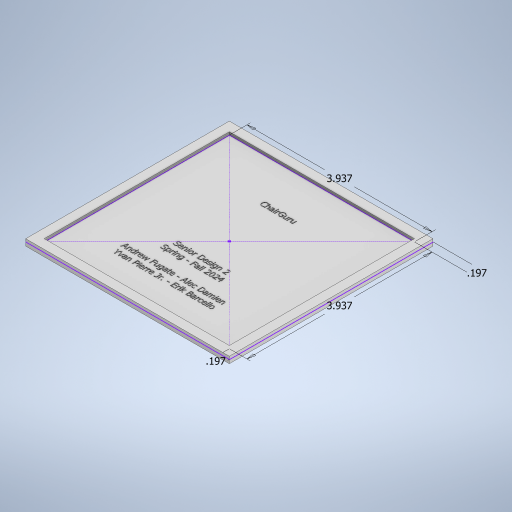
# Autodesk Inventor part: BumperCustomPCB
Saved by Autodesk Inventor 2023 (Build 270158000, 158)
## iProperties
Created: 2024-11-15
Part Number: BumperCustomPCB
Material: Generic
Document SubType Name: Modeling
Designer: andre
Density: 1 g/cm^3
Appearance: Default
Author: andre
Autodesk Inventor part; units mm, degrees
(part 1 of 3)
ref_plane "YZ Plane" through (0, 0, 0) normal (1, 0, 0) x (0, 1, 0)
ref_plane "XZ Plane" through (0, 0, 0) normal (0, 1, 0) x (-1, 0, 0)
ref_plane "XY Plane" through (0, 0, 0) normal (0, 0, 1) x (1, 0, 0)
sketch "Sketch1" plane through (0, 0, 0) normal (0, 1, 0) x (-1, 0, 0)
  line L0 (50, 50) -> (-50, 50)
  line L1 (-50, 50) -> (-50, -50)
  line L2 (-50, -50) -> (50, -50)
  line L3 (50, -50) -> (50, 50)
  line L4 (50, 50) -> (-50, -50) construction
  line L5 (-50, 50) -> (50, -50) construction
  line L6 (55, 55) -> (-55, 55)
  line L7 (-55, 55) -> (-55, -55)
  line L8 (-55, -55) -> (55, -55)
  line L9 (55, -55) -> (55, 55)
  line L10 (55, 55) -> (-55, -55) construction
  line L11 (-55, 55) -> (55, -55) construction
  point P0 (0, 0)
  dimension "d1" = 100
  dimension "d2" = 100
  dimension "d3" = 5
  dimension "d4" = 5
  constraints: 24 end point, 4 midpoint, 4 parallel, 2 horizontal, 2 perpendicular
  measures "d1" distance of L2.end L1.end
  measures "d2" distance of L1.end L0.end
  measures "d3" distance between parallel lines of L2 L8
  measures "d4" distance between parallel lines of L7 L1
extrude "Extrusion1" add sketch "Sketch1" against normal blind 2 contours L3 L2 L1 L0
extrude "Extrusion4" add sketch "Sketch1" along normal blind 1.5
extrude "Extrusion5" add sketch "Sketch1" against normal blind 2 contours L3 L2 L1 L0 | L9 L8 L7 L6
sketch "Sketch2" plane through (0, 0, 0) normal (0, 1, 0) x (1, 0, 0)
  line L0 (-9.5845, 43.6431) -> (8.9233, 43.6431) construction
  line L1 (8.9233, 43.6431) -> (8.9233, 10.4968) construction
  line L2 (8.9233, 10.4968) -> (-9.5845, 10.4968) construction
  line L3 (-9.5845, 10.4968) -> (-9.5845, 43.6431) construction
  line L4 (-49.3127, 0.1016) -> (49.3774, 0.1016) construction
  line L5 (49.3774, 0.1016) -> (49.3774, -49.8419) construction
  line L6 (49.3774, -49.8419) -> (-49.3127, -49.8419) construction
  line L7 (-49.3127, -49.8419) -> (-49.3127, 0.1016) construction
  spline S0 degree 2 poles (-8.0852, 25.4558) (-8.3816, 25.4558) (-8.883, 25.6559) (-9.0658, 25.856) knots 0 0 0 1 2 2 2
  spline S1 degree 2 poles (-9.0658, 25.856) (-9.2486, 26.0536) (-9.4486, 26.6464) (-9.4486, 27.0317) knots 0 0 0 1 2 2 2
  spline S2 degree 2 poles (-9.4486, 27.0317) (-9.4486, 27.4145) (-9.2535, 27.9826) (-9.0683, 28.1926) knots 0 0 0 1 2 2 2
  spline S3 degree 2 poles (-9.0683, 28.1926) (-8.8855, 28.3976) (-8.3865, 28.6125) (-8.0778, 28.6125) knots 0 0 0 1 2 2 2
  spline S4 degree 2 poles (-8.0778, 28.6125) (-7.9246, 28.6125) (-7.6554, 28.568) (-7.5418, 28.5335) knots 0 0 0 1 2 2 2
  spline S5 degree 2 poles (-7.5418, 28.5335) (-7.443, 28.5013) (-7.238, 28.41) (-7.1367, 28.3556) knots 0 0 0 1 2 2 2
  line L8 (-7.1367, 28.3556) -> (-7.1367, 27.8666)
  line L9 (-7.1367, 27.8666) -> (-7.1688, 27.8666)
  spline S6 degree 2 poles (-7.1688, 27.8666) (-7.2231, 27.916) (-7.3911, 28.0543) (-7.5121, 28.121) knots 0 0 0 1 2 2 2
  spline S7 degree 2 poles (-7.5121, 28.121) (-7.6282, 28.1852) (-7.9024, 28.2667) (-8.0802, 28.2667) knots 0 0 0 1 2 2 2
  spline S8 degree 2 poles (-8.0802, 28.2667) (-8.2754, 28.2667) (-8.6236, 28.1061) (-8.7546, 27.953) knots 0 0 0 1 2 2 2
  spline S9 degree 2 poles (-8.7546, 27.953) (-8.883, 27.7974) (-9.0263, 27.3256) (-9.0263, 27.0317) knots 0 0 0 1 2 2 2
  spline S10 degree 2 poles (-9.0263, 27.0317) (-9.0263, 26.718) (-8.8756, 26.266) (-8.7447, 26.1104) knots 0 0 0 1 2 2 2
  spline S11 degree 2 poles (-8.7447, 26.1104) (-8.6162, 25.9597) (-8.2729, 25.8066) (-8.0802, 25.8066) knots 0 0 0 1 2 2 2
  spline S12 degree 2 poles (-8.0802, 25.8066) (-7.9049, 25.8066) (-7.606, 25.893) (-7.4899, 25.9572) knots 0 0 0 1 2 2 2
  spline S13 degree 2 poles (-7.4899, 25.9572) (-7.3788, 26.0215) (-7.2133, 26.1548) (-7.1663, 26.2018) knots 0 0 0 1 2 2 2
  line L10 (-7.1663, 26.2018) -> (-7.1367, 26.2018)
  line L11 (-7.1367, 26.2018) -> (-7.1367, 25.7176)
  spline S14 degree 2 poles (-7.1367, 25.7176) (-7.238, 25.6707) (-7.4158, 25.5843) (-7.5418, 25.5447) knots 0 0 0 1 2 2 2
  spline S15 degree 2 poles (-7.5418, 25.5447) (-7.6752, 25.5003) (-7.9024, 25.4558) (-8.0852, 25.4558) knots 0 0 0 1 2 2 2
  line L12 (-4.9927, 25.5102) -> (-5.378, 25.5102)
  line L13 (-5.378, 25.5102) -> (-5.378, 26.8143)
  spline S16 degree 2 poles (-5.378, 26.8143) (-5.378, 26.9724) (-5.4077, 27.2441) (-5.4521, 27.3256) knots 0 0 0 1 2 2 2
  spline S17 degree 2 poles (-5.4521, 27.3256) (-5.4991, 27.4121) (-5.667, 27.4961) (-5.8103, 27.4961) knots 0 0 0 1 2 2 2
  spline S18 degree 2 poles (-5.8103, 27.4961) (-5.9536, 27.4961) (-6.2574, 27.3429) (-6.4031, 27.2194) knots 0 0 0 1 2 2 2
  line L14 (-6.4031, 27.2194) -> (-6.4031, 25.5102)
  line L15 (-6.4031, 25.5102) -> (-6.7884, 25.5102)
  line L16 (-6.7884, 25.5102) -> (-6.7884, 28.694)
  line L17 (-6.7884, 28.694) -> (-6.4031, 28.694)
  line L18 (-6.4031, 28.694) -> (-6.4031, 27.543)
  spline S19 degree 2 poles (-6.4031, 27.543) (-6.2302, 27.6986) (-5.8968, 27.8616) (-5.709, 27.8616) knots 0 0 0 1 2 2 2
  spline S20 degree 2 poles (-5.709, 27.8616) (-5.3731, 27.8616) (-4.9927, 27.417) (-4.9927, 26.9946) knots 0 0 0 1 2 2 2
  line L19 (-4.9927, 26.9946) -> (-4.9927, 25.5102)
  spline S21 degree 2 poles (-3.1773, 25.7522) (-3.2242, 25.7176) (-3.3823, 25.5941) (-3.4564, 25.5571) knots 0 0 0 1 2 2 2
  spline S22 degree 2 poles (-3.4564, 25.5571) (-3.5576, 25.5027) (-3.7478, 25.4459) (-3.9207, 25.4459) knots 0 0 0 1 2 2 2
  spline S23 degree 2 poles (-3.9207, 25.4459) (-4.0615, 25.4459) (-4.3159, 25.5521) (-4.4123, 25.6485) knots 0 0 0 1 2 2 2
  spline S24 degree 2 poles (-4.4123, 25.6485) (-4.5037, 25.7423) (-4.6148, 26.019) (-4.6148, 26.1721) knots 0 0 0 1 2 2 2
  spline S25 degree 2 poles (-4.6148, 26.1721) (-4.6148, 26.4092) (-4.4147, 26.7452) (-4.1974, 26.8415) knots 0 0 0 1 2 2 2
  spline S26 degree 2 poles (-4.1974, 26.8415) (-4.0047, 26.9304) (-3.4811, 26.9971) (-3.1773, 27.0144) knots 0 0 0 1 2 2 2
  line L20 (-3.1773, 27.0144) -> (-3.1773, 27.0885)
  spline S27 degree 2 poles (-3.1773, 27.0885) (-3.1773, 27.2219) (-3.2588, 27.3874) (-3.3329, 27.4343) knots 0 0 0 1 2 2 2
  spline S28 degree 2 poles (-3.3329, 27.4343) (-3.407, 27.4812) (-3.6194, 27.5109) (-3.733, 27.5109) knots 0 0 0 1 2 2 2
  spline S29 degree 2 poles (-3.733, 27.5109) (-3.8664, 27.5109) (-4.227, 27.4318) (-4.4073, 27.3553) knots 0 0 0 1 2 2 2
  line L21 (-4.4073, 27.3553) -> (-4.4296, 27.3553)
  line L22 (-4.4296, 27.3553) -> (-4.4296, 27.748)
  spline S30 degree 2 poles (-4.4296, 27.748) (-4.3234, 27.7776) (-3.9257, 27.8517) (-3.7305, 27.8517) knots 0 0 0 1 2 2 2
  spline S31 degree 2 poles (-3.7305, 27.8517) (-3.4934, 27.8517) (-3.1699, 27.7776) (-3.0414, 27.6813) knots 0 0 0 1 2 2 2
  spline S32 degree 2 poles (-3.0414, 27.6813) (-2.9154, 27.5874) (-2.7919, 27.2886) (-2.7919, 27.0737) knots 0 0 0 1 2 2 2
  line L23 (-2.7919, 27.0737) -> (-2.7919, 25.5102)
  line L24 (-2.7919, 25.5102) -> (-3.1773, 25.5102)
  line L25 (-3.1773, 25.5102) -> (-3.1773, 25.7522)
  line L26 (-3.1773, 26.0733) -> (-3.1773, 26.7081)
  spline S33 degree 2 poles (-3.1773, 26.7081) (-3.3156, 26.6958) (-3.733, 26.6538) (-3.8639, 26.6143) knots 0 0 0 1 2 2 2
  spline S34 degree 2 poles (-3.8639, 26.6143) (-4.0171, 26.5673) (-4.2171, 26.3722) (-4.2171, 26.1993) knots 0 0 0 1 2 2 2
  spline S35 degree 2 poles (-4.2171, 26.1993) (-4.2171, 26.0017) (-3.9948, 25.8016) (-3.7824, 25.8016) knots 0 0 0 1 2 2 2
  spline S36 degree 2 poles (-3.7824, 25.8016) (-3.6021, 25.8016) (-3.3057, 25.9572) (-3.1773, 26.0733) knots 0 0 0 1 2 2 2
  line L27 (-1.8583, 25.5102) -> (-2.2436, 25.5102)
  line L28 (-2.2436, 25.5102) -> (-2.2436, 27.7974)
  line L29 (-2.2436, 27.7974) -> (-1.8583, 27.7974)
  line L30 (-1.8583, 27.7974) -> (-1.8583, 25.5102)
  line L31 (-1.8311, 28.1778) -> (-2.2683, 28.1778)
  line L32 (-2.2683, 28.1778) -> (-2.2683, 28.5779)
  line L33 (-2.2683, 28.5779) -> (-1.8311, 28.5779)
  line L34 (-1.8311, 28.5779) -> (-1.8311, 28.1778)
  line L35 (-0.0799, 27.3849) -> (-0.0996, 27.3849)
  spline S37 degree 2 poles (-0.0996, 27.3849) (-0.1441, 27.3973) (-0.2404, 27.4022) (-0.3071, 27.4022) knots 0 0 0 1 2 2 2
  spline S38 degree 2 poles (-0.3071, 27.4022) (-0.4627, 27.4022) (-0.769, 27.2663) (-0.9073, 27.133) knots 0 0 0 1 2 2 2
  line L36 (-0.9073, 27.133) -> (-0.9073, 25.5102)
  line L37 (-0.9073, 25.5102) -> (-1.2926, 25.5102)
  line L38 (-1.2926, 25.5102) -> (-1.2926, 27.7974)
  line L39 (-1.2926, 27.7974) -> (-0.9073, 27.7974)
  line L40 (-0.9073, 27.7974) -> (-0.9073, 27.4565)
  spline S39 degree 2 poles (-0.9073, 27.4565) (-0.6974, 27.6443) (-0.3837, 27.7974) (-0.2355, 27.7974) knots 0 0 0 1 2 2 2
  spline S40 degree 2 poles (-0.2355, 27.7974) (-0.1762, 27.7974) (-0.1169, 27.7925) (-0.0799, 27.785) knots 0 0 0 1 2 2 2
  line L41 (-0.0799, 27.785) -> (-0.0799, 27.3849)
  spline S41 degree 2 poles (1.5256, 25.4509) (1.2021, 25.4509) (0.6661, 25.6485) (0.4734, 25.8486) knots 0 0 0 1 2 2 2
  spline S42 degree 2 poles (0.4734, 25.8486) (0.2808, 26.0511) (0.0757, 26.6488) (0.0757, 27.0366) knots 0 0 0 1 2 2 2
  spline S43 degree 2 poles (0.0757, 27.0366) (0.0757, 27.4047) (0.2832, 27.9876) (0.4759, 28.1951) knots 0 0 0 1 2 2 2
  spline S44 degree 2 poles (0.4759, 28.1951) (0.6611, 28.3951) (1.2045, 28.6125) (1.5281, 28.6125) knots 0 0 0 1 2 2 2
  spline S45 degree 2 poles (1.5281, 28.6125) (1.6837, 28.6125) (1.9653, 28.568) (2.0938, 28.5285) knots 0 0 0 1 2 2 2
  spline S46 degree 2 poles (2.0938, 28.5285) (2.1975, 28.4989) (2.4494, 28.3902) (2.526, 28.3507) knots 0 0 0 1 2 2 2
  line L42 (2.526, 28.3507) -> (2.526, 27.8616)
  line L43 (2.526, 27.8616) -> (2.4914, 27.8616)
  spline S47 degree 2 poles (2.4914, 27.8616) (2.4149, 27.9283) (2.2543, 28.0493) (2.1061, 28.1185) knots 0 0 0 1 2 2 2
  spline S48 degree 2 poles (2.1061, 28.1185) (1.9826, 28.1802) (1.664, 28.2618) (1.4812, 28.2618) knots 0 0 0 1 2 2 2
  spline S49 degree 2 poles (1.4812, 28.2618) (1.0415, 28.2618) (0.4981, 27.5998) (0.4981, 27.049) knots 0 0 0 1 2 2 2
  spline S50 degree 2 poles (0.4981, 27.049) (0.4981, 26.7427) (0.6414, 26.2833) (0.7772, 26.1252) knots 0 0 0 1 2 2 2
  spline S51 degree 2 poles (0.7772, 26.1252) (0.9081, 25.9671) (1.2786, 25.8016) (1.5108, 25.8016) knots 0 0 0 1 2 2 2
  spline S52 degree 2 poles (1.5108, 25.8016) (1.6813, 25.8016) (2.0221, 25.851) (2.1382, 25.9004) knots 0 0 0 1 2 2 2
  line L44 (2.1382, 25.9004) -> (2.1382, 26.6884)
  line L45 (2.1382, 26.6884) -> (1.4318, 26.6884)
  line L46 (1.4318, 26.6884) -> (1.4318, 27.044)
  line L47 (1.4318, 27.044) -> (2.5384, 27.044)
  line L48 (2.5384, 27.044) -> (2.5384, 25.7127)
  spline S53 degree 2 poles (2.5384, 25.7127) (2.4618, 25.6781) (2.2, 25.5719) (2.0888, 25.5398) knots 0 0 0 1 2 2 2
  spline S54 degree 2 poles (2.0888, 25.5398) (1.9381, 25.4953) (1.6961, 25.4509) (1.5256, 25.4509) knots 0 0 0 1 2 2 2
  line L49 (4.7959, 25.5102) -> (4.4106, 25.5102)
  line L50 (4.4106, 25.5102) -> (4.4106, 25.7621)
  spline S55 degree 2 poles (4.4106, 25.7621) (4.2328, 25.6065) (3.9142, 25.4459) (3.7166, 25.4459) knots 0 0 0 1 2 2 2
  spline S56 degree 2 poles (3.7166, 25.4459) (3.5684, 25.4459) (3.3041, 25.5447) (3.2077, 25.6509) knots 0 0 0 1 2 2 2
  spline S57 degree 2 poles (3.2077, 25.6509) (3.1089, 25.7572) (3.0002, 26.0807) (3.0002, 26.3129) knots 0 0 0 1 2 2 2
  line L51 (3.0002, 26.3129) -> (3.0002, 27.7974)
  line L52 (3.0002, 27.7974) -> (3.3856, 27.7974)
  line L53 (3.3856, 27.7974) -> (3.3856, 26.4932)
  spline S58 degree 2 poles (3.3856, 26.4932) (3.3856, 26.3104) (3.4127, 26.0709) (3.4597, 25.9819) knots 0 0 0 1 2 2 2
  spline S59 degree 2 poles (3.4597, 25.9819) (3.5066, 25.893) (3.6672, 25.8115) (3.8178, 25.8115) knots 0 0 0 1 2 2 2
  spline S60 degree 2 poles (3.8178, 25.8115) (3.9586, 25.8115) (4.2772, 25.9721) (4.4106, 26.0881) knots 0 0 0 1 2 2 2
  line L54 (4.4106, 26.0881) -> (4.4106, 27.7974)
  line L55 (4.4106, 27.7974) -> (4.7959, 27.7974)
  line L56 (4.7959, 27.7974) -> (4.7959, 25.5102)
  line L57 (6.567, 27.3849) -> (6.5472, 27.3849)
  spline S61 degree 2 poles (6.5472, 27.3849) (6.5027, 27.3973) (6.4064, 27.4022) (6.3397, 27.4022) knots 0 0 0 1 2 2 2
  spline S62 degree 2 poles (6.3397, 27.4022) (6.1841, 27.4022) (5.8778, 27.2663) (5.7395, 27.133) knots 0 0 0 1 2 2 2
  line L58 (5.7395, 27.133) -> (5.7395, 25.5102)
  line L59 (5.7395, 25.5102) -> (5.3542, 25.5102)
  line L60 (5.3542, 25.5102) -> (5.3542, 27.7974)
  line L61 (5.3542, 27.7974) -> (5.7395, 27.7974)
  line L62 (5.7395, 27.7974) -> (5.7395, 27.4565)
  spline S63 degree 2 poles (5.7395, 27.4565) (5.9494, 27.6443) (6.2631, 27.7974) (6.4113, 27.7974) knots 0 0 0 1 2 2 2
  spline S64 degree 2 poles (6.4113, 27.7974) (6.4706, 27.7974) (6.5299, 27.7925) (6.567, 27.785) knots 0 0 0 1 2 2 2
  line L63 (6.567, 27.785) -> (6.567, 27.3849)
  line L64 (8.6442, 25.5102) -> (8.2589, 25.5102)
  line L65 (8.2589, 25.5102) -> (8.2589, 25.7621)
  spline S65 degree 2 poles (8.2589, 25.7621) (8.0811, 25.6065) (7.7624, 25.4459) (7.5648, 25.4459) knots 0 0 0 1 2 2 2
  spline S66 degree 2 poles (7.5648, 25.4459) (7.4166, 25.4459) (7.1523, 25.5447) (7.056, 25.6509) knots 0 0 0 1 2 2 2
  spline S67 degree 2 poles (7.056, 25.6509) (6.9572, 25.7572) (6.8485, 26.0807) (6.8485, 26.3129) knots 0 0 0 1 2 2 2
  line L66 (6.8485, 26.3129) -> (6.8485, 27.7974)
  line L67 (6.8485, 27.7974) -> (7.2339, 27.7974)
  line L68 (7.2339, 27.7974) -> (7.2339, 26.4932)
  spline S68 degree 2 poles (7.2339, 26.4932) (7.2339, 26.3104) (7.261, 26.0709) (7.308, 25.9819) knots 0 0 0 1 2 2 2
  spline S69 degree 2 poles (7.308, 25.9819) (7.3549, 25.893) (7.5154, 25.8115) (7.6661, 25.8115) knots 0 0 0 1 2 2 2
  spline S70 degree 2 poles (7.6661, 25.8115) (7.8069, 25.8115) (8.1255, 25.9721) (8.2589, 26.0881) knots 0 0 0 1 2 2 2
  line L69 (8.2589, 26.0881) -> (8.2589, 27.7974)
  line L70 (8.2589, 27.7974) -> (8.6442, 27.7974)
  line L71 (8.6442, 27.7974) -> (8.6442, 25.5102)
  spline S71 degree 2 poles (-13.3379, -16.4116) (-13.6688, -16.4116) (-14.1332, -16.2733) (-14.3382, -16.1745) knots 0 0 0 1 2 2 2
  line L72 (-14.3382, -16.1745) -> (-14.3382, -15.6657)
  line L73 (-14.3382, -15.6657) -> (-14.3086, -15.6657)
  spline S72 degree 2 poles (-14.3086, -15.6657) (-14.1085, -15.8534) (-13.6022, -16.0609) (-13.3675, -16.0609) knots 0 0 0 1 2 2 2
  spline S73 degree 2 poles (-13.3675, -16.0609) (-13.0316, -16.0609) (-12.6882, -15.7818) (-12.6882, -15.552) knots 0 0 0 1 2 2 2
  spline S74 degree 2 poles (-12.6882, -15.552) (-12.6882, -15.3693) (-12.8686, -15.142) (-13.0637, -15.0852) knots 0 0 0 1 2 2 2
  spline S75 degree 2 poles (-13.0637, -15.0852) (-13.2045, -15.0457) (-13.4391, -14.9914) (-13.6145, -14.9469) knots 0 0 0 1 2 2 2
  spline S76 degree 2 poles (-13.6145, -14.9469) (-13.7726, -14.9049) (-14.0221, -14.7789) (-14.1184, -14.6777) knots 0 0 0 1 2 2 2
  spline S77 degree 2 poles (-14.1184, -14.6777) (-14.2122, -14.5764) (-14.316, -14.3047) (-14.316, -14.1268) knots 0 0 0 1 2 2 2
  spline S78 degree 2 poles (-14.316, -14.1268) (-14.316, -13.7563) (-13.738, -13.2549) (-13.2909, -13.2549) knots 0 0 0 1 2 2 2
  spline S79 degree 2 poles (-13.2909, -13.2549) (-13.0341, -13.2549) (-12.5796, -13.3562) (-12.3844, -13.4525) knots 0 0 0 1 2 2 2
  line L74 (-12.3844, -13.4525) -> (-12.3844, -13.9367)
  line L75 (-12.3844, -13.9367) -> (-12.4141, -13.9367)
  spline S80 degree 2 poles (-12.4141, -13.9367) (-12.5598, -13.8033) (-13.0143, -13.6057) (-13.2638, -13.6057) knots 0 0 0 1 2 2 2
  spline S81 degree 2 poles (-13.2638, -13.6057) (-13.5453, -13.6057) (-13.8936, -13.87) (-13.8936, -14.0849) knots 0 0 0 1 2 2 2
  spline S82 degree 2 poles (-13.8936, -14.0849) (-13.8936, -14.2775) (-13.6886, -14.5072) (-13.4959, -14.5591) knots 0 0 0 1 2 2 2
  spline S83 degree 2 poles (-13.4959, -14.5591) (-13.3675, -14.5937) (-12.9945, -14.6826) (-12.871, -14.7197) knots 0 0 0 1 2 2 2
  spline S84 degree 2 poles (-12.871, -14.7197) (-12.5573, -14.816) (-12.2659, -15.2038) (-12.2659, -15.4878) knots 0 0 0 1 2 2 2
  spline S85 degree 2 poles (-12.2659, -15.4878) (-12.2659, -15.6681) (-12.4116, -16.0139) (-12.5425, -16.135) knots 0 0 0 1 2 2 2
  spline S86 degree 2 poles (-12.5425, -16.135) (-12.6882, -16.2684) (-13.0588, -16.4116) (-13.3379, -16.4116) knots 0 0 0 1 2 2 2
  spline S87 degree 2 poles (-10.8901, -16.4091) (-11.4384, -16.4091) (-12.0411, -15.7941) (-12.0411, -15.226) knots 0 0 0 1 2 2 2
  spline S88 degree 2 poles (-12.0411, -15.226) (-12.0411, -14.6678) (-11.4557, -14.0058) (-10.9839, -14.0058) knots 0 0 0 1 2 2 2
  spline S89 degree 2 poles (-10.9839, -14.0058) (-10.7715, -14.0058) (-10.443, -14.1293) (-10.322, -14.2602) knots 0 0 0 1 2 2 2
  spline S90 degree 2 poles (-10.322, -14.2602) (-10.1985, -14.3911) (-10.0676, -14.7691) (-10.0676, -15.0432) knots 0 0 0 1 2 2 2
  line L76 (-10.0676, -15.0432) -> (-10.0676, -15.2532)
  line L77 (-10.0676, -15.2532) -> (-11.6508, -15.2532)
  spline S91 degree 2 poles (-11.6508, -15.2532) (-11.6508, -15.6508) (-11.2507, -16.0732) (-10.895, -16.0732) knots 0 0 0 1 2 2 2
  spline S92 degree 2 poles (-10.895, -16.0732) (-10.769, -16.0732) (-10.5245, -16.0164) (-10.4257, -15.972) knots 0 0 0 1 2 2 2
  spline S93 degree 2 poles (-10.4257, -15.972) (-10.322, -15.9226) (-10.1787, -15.8361) (-10.1318, -15.7966) knots 0 0 0 1 2 2 2
  line L78 (-10.1318, -15.7966) -> (-10.1096, -15.7966)
  line L79 (-10.1096, -15.7966) -> (-10.1096, -16.2165)
  spline S94 degree 2 poles (-10.1096, -16.2165) (-10.1762, -16.2437) (-10.3788, -16.3227) (-10.4578, -16.3449) knots 0 0 0 1 2 2 2
  spline S95 degree 2 poles (-10.4578, -16.3449) (-10.569, -16.377) (-10.7518, -16.4091) (-10.8901, -16.4091) knots 0 0 0 1 2 2 2
  spline S96 degree 2 poles (-10.443, -14.9592) (-10.4479, -14.8036) (-10.5122, -14.5764) (-10.5739, -14.4998) knots 0 0 0 1 2 2 2
  spline S97 degree 2 poles (-10.5739, -14.4998) (-10.6406, -14.4134) (-10.8506, -14.322) (-11.0062, -14.322) knots 0 0 0 1 2 2 2
  spline S98 degree 2 poles (-11.0062, -14.322) (-11.1593, -14.322) (-11.3742, -14.4134) (-11.4631, -14.5023) knots 0 0 0 1 2 2 2
  spline S99 degree 2 poles (-11.4631, -14.5023) (-11.5496, -14.5937) (-11.6385, -14.8135) (-11.6508, -14.9592) knots 0 0 0 1 2 2 2
  line L80 (-11.6508, -14.9592) -> (-10.443, -14.9592)
  line L81 (-7.8816, -16.3573) -> (-8.2669, -16.3573)
  line L82 (-8.2669, -16.3573) -> (-8.2669, -15.0531)
  spline S100 degree 2 poles (-8.2669, -15.0531) (-8.2669, -14.895) (-8.2966, -14.6233) (-8.341, -14.5418) knots 0 0 0 1 2 2 2
  spline S101 degree 2 poles (-8.341, -14.5418) (-8.388, -14.4554) (-8.5559, -14.3714) (-8.6992, -14.3714) knots 0 0 0 1 2 2 2
  spline S102 degree 2 poles (-8.6992, -14.3714) (-8.8424, -14.3714) (-9.1462, -14.5245) (-9.292, -14.648) knots 0 0 0 1 2 2 2
  line L83 (-9.292, -14.648) -> (-9.292, -16.3573)
  line L84 (-9.292, -16.3573) -> (-9.6773, -16.3573)
  line L85 (-9.6773, -16.3573) -> (-9.6773, -14.07)
  line L86 (-9.6773, -14.07) -> (-9.292, -14.07)
  line L87 (-9.292, -14.07) -> (-9.292, -14.3244)
  spline S103 degree 2 poles (-9.292, -14.3244) (-9.1191, -14.1688) (-8.7856, -14.0058) (-8.5979, -14.0058) knots 0 0 0 1 2 2 2
  spline S104 degree 2 poles (-8.5979, -14.0058) (-8.262, -14.0058) (-7.8816, -14.4504) (-7.8816, -14.8728) knots 0 0 0 1 2 2 2
  line L88 (-7.8816, -14.8728) -> (-7.8816, -16.3573)
  line L89 (-6.9479, -16.3573) -> (-7.3333, -16.3573)
  line L90 (-7.3333, -16.3573) -> (-7.3333, -14.07)
  line L91 (-7.3333, -14.07) -> (-6.9479, -14.07)
  line L92 (-6.9479, -14.07) -> (-6.9479, -16.3573)
  line L93 (-6.9208, -13.6897) -> (-7.358, -13.6897)
  line L94 (-7.358, -13.6897) -> (-7.358, -13.2895)
  line L95 (-7.358, -13.2895) -> (-6.9208, -13.2895)
  line L96 (-6.9208, -13.2895) -> (-6.9208, -13.6897)
  spline S105 degree 2 poles (-4.5026, -15.2137) (-4.5026, -15.7916) (-5.0584, -16.4215) (-5.5227, -16.4215) knots 0 0 0 1 2 2 2
  spline S106 degree 2 poles (-5.5227, -16.4215) (-5.9994, -16.4215) (-6.5453, -15.7719) (-6.5453, -15.2137) knots 0 0 0 1 2 2 2
  spline S107 degree 2 poles (-6.5453, -15.2137) (-6.5453, -14.6406) (-5.9822, -14.0058) (-5.5227, -14.0058) knots 0 0 0 1 2 2 2
  spline S108 degree 2 poles (-5.5227, -14.0058) (-5.0584, -14.0058) (-4.5026, -14.6381) (-4.5026, -15.2137) knots 0 0 0 1 2 2 2
  spline S109 degree 2 poles (-4.9003, -15.2137) (-4.9003, -14.7691) (-5.2239, -14.3368) (-5.5227, -14.3368) knots 0 0 0 1 2 2 2
  spline S110 degree 2 poles (-5.5227, -14.3368) (-5.8216, -14.3368) (-6.1476, -14.7691) (-6.1476, -15.2137) knots 0 0 0 1 2 2 2
  spline S111 degree 2 poles (-6.1476, -15.2137) (-6.1476, -15.6459) (-5.8216, -16.0905) (-5.5227, -16.0905) knots 0 0 0 1 2 2 2
  spline S112 degree 2 poles (-5.5227, -16.0905) (-5.2263, -16.0905) (-4.9003, -15.6533) (-4.9003, -15.2137) knots 0 0 0 1 2 2 2
  line L97 (-2.8946, -14.4825) -> (-2.9144, -14.4825)
  spline S113 degree 2 poles (-2.9144, -14.4825) (-2.9589, -14.4702) (-3.0552, -14.4652) (-3.1219, -14.4652) knots 0 0 0 1 2 2 2
  spline S114 degree 2 poles (-3.1219, -14.4652) (-3.2775, -14.4652) (-3.5838, -14.6011) (-3.7221, -14.7345) knots 0 0 0 1 2 2 2
  line L98 (-3.7221, -14.7345) -> (-3.7221, -16.3573)
  line L99 (-3.7221, -16.3573) -> (-4.1074, -16.3573)
  line L100 (-4.1074, -16.3573) -> (-4.1074, -14.07)
  line L101 (-4.1074, -14.07) -> (-3.7221, -14.07)
  line L102 (-3.7221, -14.07) -> (-3.7221, -14.4109)
  spline S115 degree 2 poles (-3.7221, -14.4109) (-3.5121, -14.2232) (-3.1984, -14.07) (-3.0502, -14.07) knots 0 0 0 1 2 2 2
  spline S116 degree 2 poles (-3.0502, -14.07) (-2.991, -14.07) (-2.9317, -14.075) (-2.8946, -14.0824) knots 0 0 0 1 2 2 2
  line L103 (-2.8946, -14.0824) -> (-2.8946, -14.4825)
  spline S117 degree 2 poles (1.1463, -14.8357) (1.1463, -15.2532) (0.8079, -15.925) (0.5239, -16.1127) knots 0 0 0 1 2 2 2
  spline S118 degree 2 poles (0.5239, -16.1127) (0.2917, -16.2585) (-0.185, -16.3573) (-0.5555, -16.3573) knots 0 0 0 1 2 2 2
  line L104 (-0.5555, -16.3573) -> (-1.257, -16.3573)
  line L105 (-1.257, -16.3573) -> (-1.257, -13.3093)
  line L106 (-1.257, -13.3093) -> (-0.5629, -13.3093)
  spline S119 degree 2 poles (-0.5629, -13.3093) (-0.1332, -13.3093) (0.3559, -13.4377) (0.5288, -13.5513) knots 0 0 0 1 2 2 2
  spline S120 degree 2 poles (0.5288, -13.5513) (0.8227, -13.7465) (1.1463, -14.3911) (1.1463, -14.8357) knots 0 0 0 1 2 2 2
  spline S121 degree 2 poles (0.7239, -14.8308) (0.7239, -14.4801) (0.4918, -13.9836) (0.262, -13.8428) knots 0 0 0 1 2 2 2
  spline S122 degree 2 poles (0.262, -13.8428) (0.099, -13.7465) (-0.269, -13.66) (-0.5432, -13.66) knots 0 0 0 1 2 2 2
  line L107 (-0.5432, -13.66) -> (-0.8519, -13.66)
  line L108 (-0.8519, -13.66) -> (-0.8519, -16.0065)
  line L109 (-0.8519, -16.0065) -> (-0.5432, -16.0065)
  spline S123 degree 2 poles (-0.5432, -16.0065) (-0.2739, -16.0065) (0.1336, -15.9201) (0.2991, -15.804) knots 0 0 0 1 2 2 2
  spline S124 degree 2 poles (0.2991, -15.804) (0.5115, -15.6607) (0.7239, -15.1865) (0.7239, -14.8308) knots 0 0 0 1 2 2 2
  spline S125 degree 2 poles (2.5493, -16.4091) (2.0009, -16.4091) (1.3983, -15.7941) (1.3983, -15.226) knots 0 0 0 1 2 2 2
  spline S126 degree 2 poles (1.3983, -15.226) (1.3983, -14.6678) (1.9836, -14.0058) (2.4554, -14.0058) knots 0 0 0 1 2 2 2
  spline S127 degree 2 poles (2.4554, -14.0058) (2.6678, -14.0058) (2.9964, -14.1293) (3.1174, -14.2602) knots 0 0 0 1 2 2 2
  spline S128 degree 2 poles (3.1174, -14.2602) (3.2409, -14.3911) (3.3718, -14.7691) (3.3718, -15.0432) knots 0 0 0 1 2 2 2
  line L110 (3.3718, -15.0432) -> (3.3718, -15.2532)
  line L111 (3.3718, -15.2532) -> (1.7885, -15.2532)
  spline S129 degree 2 poles (1.7885, -15.2532) (1.7885, -15.6508) (2.1887, -16.0732) (2.5443, -16.0732) knots 0 0 0 1 2 2 2
  spline S130 degree 2 poles (2.5443, -16.0732) (2.6703, -16.0732) (2.9148, -16.0164) (3.0136, -15.972) knots 0 0 0 1 2 2 2
  spline S131 degree 2 poles (3.0136, -15.972) (3.1174, -15.9226) (3.2606, -15.8361) (3.3076, -15.7966) knots 0 0 0 1 2 2 2
  line L112 (3.3076, -15.7966) -> (3.3298, -15.7966)
  line L113 (3.3298, -15.7966) -> (3.3298, -16.2165)
  spline S132 degree 2 poles (3.3298, -16.2165) (3.2631, -16.2437) (3.0606, -16.3227) (2.9815, -16.3449) knots 0 0 0 1 2 2 2
  spline S133 degree 2 poles (2.9815, -16.3449) (2.8704, -16.377) (2.6876, -16.4091) (2.5493, -16.4091) knots 0 0 0 1 2 2 2
  spline S134 degree 2 poles (2.9964, -14.9592) (2.9914, -14.8036) (2.9272, -14.5764) (2.8654, -14.4998) knots 0 0 0 1 2 2 2
  spline S135 degree 2 poles (2.8654, -14.4998) (2.7988, -14.4134) (2.5888, -14.322) (2.4332, -14.322) knots 0 0 0 1 2 2 2
  spline S136 degree 2 poles (2.4332, -14.322) (2.28, -14.322) (2.0652, -14.4134) (1.9762, -14.5023) knots 0 0 0 1 2 2 2
  spline S137 degree 2 poles (1.9762, -14.5023) (1.8898, -14.5937) (1.8009, -14.8135) (1.7885, -14.9592) knots 0 0 0 1 2 2 2
  line L114 (1.7885, -14.9592) -> (2.9964, -14.9592)
  spline S138 degree 2 poles (4.3796, -16.4116) (4.1499, -16.4116) (3.7522, -16.2881) (3.6213, -16.219) knots 0 0 0 1 2 2 2
  line L115 (3.6213, -16.219) -> (3.6213, -15.7867)
  line L116 (3.6213, -15.7867) -> (3.641, -15.7867)
  spline S139 degree 2 poles (3.641, -15.7867) (3.6904, -15.8262) (3.8238, -15.9201) (3.935, -15.972) knots 0 0 0 1 2 2 2
  spline S140 degree 2 poles (3.935, -15.972) (4.0313, -16.0189) (4.2684, -16.088) (4.3944, -16.088) knots 0 0 0 1 2 2 2
  spline S141 degree 2 poles (4.3944, -16.088) (4.4858, -16.088) (4.6957, -16.0461) (4.7451, -16.0115) knots 0 0 0 1 2 2 2
  spline S142 degree 2 poles (4.7451, -16.0115) (4.8168, -15.9645) (4.881, -15.8583) (4.881, -15.7496) knots 0 0 0 1 2 2 2
  spline S143 degree 2 poles (4.881, -15.7496) (4.881, -15.6138) (4.7328, -15.473) (4.5426, -15.4261) knots 0 0 0 1 2 2 2
  spline S144 degree 2 poles (4.5426, -15.4261) (4.4685, -15.4088) (4.2314, -15.3594) (4.1301, -15.3322) knots 0 0 0 1 2 2 2
  spline S145 degree 2 poles (4.1301, -15.3322) (3.8683, -15.2556) (3.6311, -14.9395) (3.6311, -14.7147) knots 0 0 0 1 2 2 2
  spline S146 degree 2 poles (3.6311, -14.7147) (3.6311, -14.4035) (4.098, -14.0157) (4.4833, -14.0157) knots 0 0 0 1 2 2 2
  spline S147 degree 2 poles (4.4833, -14.0157) (4.6735, -14.0157) (5.0588, -14.1096) (5.1897, -14.1812) knots 0 0 0 1 2 2 2
  line L117 (5.1897, -14.1812) -> (5.1897, -14.5937)
  line L118 (5.1897, -14.5937) -> (5.17, -14.5937)
  spline S148 degree 2 poles (5.17, -14.5937) (5.0218, -14.4751) (4.6611, -14.3393) (4.4759, -14.3393) knots 0 0 0 1 2 2 2
  spline S149 degree 2 poles (4.4759, -14.3393) (4.2857, -14.3393) (4.0239, -14.4998) (4.0239, -14.6604) knots 0 0 0 1 2 2 2
  spline S150 degree 2 poles (4.0239, -14.6604) (4.0239, -14.8061) (4.1795, -14.9469) (4.3524, -14.9914) knots 0 0 0 1 2 2 2
  spline S151 degree 2 poles (4.3524, -14.9914) (4.4364, -15.0136) (4.6488, -15.058) (4.7649, -15.0852) knots 0 0 0 1 2 2 2
  spline S152 degree 2 poles (4.7649, -15.0852) (5.0168, -15.1494) (5.2737, -15.4434) (5.2737, -15.6978) knots 0 0 0 1 2 2 2
  spline S153 degree 2 poles (5.2737, -15.6978) (5.2737, -15.846) (5.1576, -16.1078) (5.044, -16.2041) knots 0 0 0 1 2 2 2
  spline S154 degree 2 poles (5.044, -16.2041) (4.923, -16.3054) (4.6142, -16.4116) (4.3796, -16.4116) knots 0 0 0 1 2 2 2
  line L119 (6.0246, -16.3573) -> (5.6393, -16.3573)
  line L120 (5.6393, -16.3573) -> (5.6393, -14.07)
  line L121 (5.6393, -14.07) -> (6.0246, -14.07)
  line L122 (6.0246, -14.07) -> (6.0246, -16.3573)
  line L123 (6.0518, -13.6897) -> (5.6146, -13.6897)
  line L124 (5.6146, -13.6897) -> (5.6146, -13.2895)
  line L125 (5.6146, -13.2895) -> (6.0518, -13.2895)
  line L126 (6.0518, -13.2895) -> (6.0518, -13.6897)
  spline S155 degree 2 poles (6.6717, -16.7228) (6.7113, -16.7401) (6.8619, -16.7945) (6.9583, -16.8167) knots 0 0 0 1 2 2 2
  spline S156 degree 2 poles (6.9583, -16.8167) (7.0645, -16.8439) (7.2448, -16.876) (7.351, -16.876) knots 0 0 0 1 2 2 2
  spline S157 degree 2 poles (7.351, -16.876) (7.5288, -16.876) (7.7758, -16.7821) (7.845, -16.6981) knots 0 0 0 1 2 2 2
  spline S158 degree 2 poles (7.845, -16.6981) (7.9117, -16.6142) (7.9636, -16.3943) (7.9636, -16.2535) knots 0 0 0 1 2 2 2
  line L127 (7.9636, -16.2535) -> (7.9636, -16.0535)
  spline S159 degree 2 poles (7.9636, -16.0535) (7.8079, -16.1893) (7.5091, -16.3178) (7.2843, -16.3178) knots 0 0 0 1 2 2 2
  spline S160 degree 2 poles (7.2843, -16.3178) (6.894, -16.3178) (6.4321, -15.7373) (6.4321, -15.1914) knots 0 0 0 1 2 2 2
  spline S161 degree 2 poles (6.4321, -15.1914) (6.4321, -14.9074) (6.5927, -14.4677) (6.7261, -14.3121) knots 0 0 0 1 2 2 2
  spline S162 degree 2 poles (6.7261, -14.3121) (6.8545, -14.1664) (7.2077, -14.0058) (7.3955, -14.0058) knots 0 0 0 1 2 2 2
  spline S163 degree 2 poles (7.3955, -14.0058) (7.5733, -14.0058) (7.8326, -14.0898) (7.9636, -14.1664) knots 0 0 0 1 2 2 2
  line L128 (7.9636, -14.1664) -> (7.9858, -14.07)
  line L129 (7.9858, -14.07) -> (8.3489, -14.07)
  line L130 (8.3489, -14.07) -> (8.3489, -16.0955)
  spline S164 degree 2 poles (8.3489, -16.0955) (8.3489, -16.6784) (7.8425, -17.2218) (7.3214, -17.2218) knots 0 0 0 1 2 2 2
  spline S165 degree 2 poles (7.3214, -17.2218) (7.1534, -17.2218) (6.8026, -17.1674) (6.652, -17.123) knots 0 0 0 1 2 2 2
  line L131 (6.652, -17.123) -> (6.652, -16.7228)
  line L132 (6.652, -16.7228) -> (6.6717, -16.7228)
  line L133 (7.9636, -15.7373) -> (7.9636, -14.4801)
  spline S166 degree 2 poles (7.9636, -14.4801) (7.8203, -14.4109) (7.5782, -14.3516) (7.4572, -14.3516) knots 0 0 0 1 2 2 2
  spline S167 degree 2 poles (7.4572, -14.3516) (7.1657, -14.3516) (6.8298, -14.7814) (6.8298, -15.184) knots 0 0 0 1 2 2 2
  spline S168 degree 2 poles (6.8298, -15.184) (6.8298, -15.5644) (7.0842, -15.9621) (7.3708, -15.9621) knots 0 0 0 1 2 2 2
  spline S169 degree 2 poles (7.3708, -15.9621) (7.5214, -15.9621) (7.8376, -15.8435) (7.9636, -15.7373) knots 0 0 0 1 2 2 2
  line L134 (10.7028, -16.3573) -> (10.3175, -16.3573)
  line L135 (10.3175, -16.3573) -> (10.3175, -15.0531)
  spline S170 degree 2 poles (10.3175, -15.0531) (10.3175, -14.895) (10.2878, -14.6233) (10.2434, -14.5418) knots 0 0 0 1 2 2 2
  spline S171 degree 2 poles (10.2434, -14.5418) (10.1965, -14.4554) (10.0285, -14.3714) (9.8852, -14.3714) knots 0 0 0 1 2 2 2
  spline S172 degree 2 poles (9.8852, -14.3714) (9.742, -14.3714) (9.4382, -14.5245) (9.2924, -14.648) knots 0 0 0 1 2 2 2
  line L136 (9.2924, -14.648) -> (9.2924, -16.3573)
  line L137 (9.2924, -16.3573) -> (8.9071, -16.3573)
  line L138 (8.9071, -16.3573) -> (8.9071, -14.07)
  line L139 (8.9071, -14.07) -> (9.2924, -14.07)
  line L140 (9.2924, -14.07) -> (9.2924, -14.3244)
  spline S173 degree 2 poles (9.2924, -14.3244) (9.4653, -14.1688) (9.7988, -14.0058) (9.9865, -14.0058) knots 0 0 0 1 2 2 2
  spline S174 degree 2 poles (9.9865, -14.0058) (10.3224, -14.0058) (10.7028, -14.4504) (10.7028, -14.8728) knots 0 0 0 1 2 2 2
  line L141 (10.7028, -14.8728) -> (10.7028, -16.3573)
  line L142 (14.3757, -16.3573) -> (12.496, -16.3573)
  line L143 (12.496, -16.3573) -> (12.496, -15.925)
  spline S175 degree 2 poles (12.496, -15.925) (12.6986, -15.7348) (13.0592, -15.3816) (13.2321, -15.1914) knots 0 0 0 1 2 2 2
  spline S176 degree 2 poles (13.2321, -15.1914) (13.5804, -14.8086) (13.8348, -14.3491) (13.8348, -14.1046) knots 0 0 0 1 2 2 2
  spline S177 degree 2 poles (13.8348, -14.1046) (13.8348, -13.9762) (13.7557, -13.7835) (13.6841, -13.7218) knots 0 0 0 1 2 2 2
  spline S178 degree 2 poles (13.6841, -13.7218) (13.6125, -13.66) (13.4248, -13.5983) (13.3111, -13.5983) knots 0 0 0 1 2 2 2
  spline S179 degree 2 poles (13.3111, -13.5983) (13.2025, -13.5983) (12.9802, -13.6526) (12.8789, -13.6946) knots 0 0 0 1 2 2 2
  spline S180 degree 2 poles (12.8789, -13.6946) (12.7924, -13.7292) (12.6319, -13.828) (12.5825, -13.8626) knots 0 0 0 1 2 2 2
  line L144 (12.5825, -13.8626) -> (12.5603, -13.8626)
  line L145 (12.5603, -13.8626) -> (12.5603, -13.4278)
  spline S181 degree 2 poles (12.5603, -13.4278) (12.6862, -13.3661) (13.1382, -13.2451) (13.3408, -13.2451) knots 0 0 0 1 2 2 2
  spline S182 degree 2 poles (13.3408, -13.2451) (13.7681, -13.2451) (14.2497, -13.6971) (14.2497, -14.0824) knots 0 0 0 1 2 2 2
  spline S183 degree 2 poles (14.2497, -14.0824) (14.2497, -14.2627) (14.1658, -14.564) (14.0917, -14.6925) knots 0 0 0 1 2 2 2
  spline S184 degree 2 poles (14.0917, -14.6925) (14.0176, -14.8259) (13.8027, -15.0877) (13.6841, -15.2137) knots 0 0 0 1 2 2 2
  spline S185 degree 2 poles (13.6841, -15.2137) (13.4915, -15.4236) (13.0197, -15.8731) (12.8789, -16.0041) knots 0 0 0 1 2 2 2
  line L146 (12.8789, -16.0041) -> (14.3757, -16.0041)
  line L147 (14.3757, -16.0041) -> (14.3757, -16.3573)
  spline S186 degree 2 poles (-15.1471, -21.4301) (-15.4781, -21.4301) (-15.9425, -21.2917) (-16.1475, -21.1929) knots 0 0 0 1 2 2 2
  line L148 (-16.1475, -21.1929) -> (-16.1475, -20.6841)
  line L149 (-16.1475, -20.6841) -> (-16.1179, -20.6841)
  spline S187 degree 2 poles (-16.1179, -20.6841) (-15.9178, -20.8718) (-15.4114, -21.0793) (-15.1768, -21.0793) knots 0 0 0 1 2 2 2
  spline S188 degree 2 poles (-15.1768, -21.0793) (-14.8409, -21.0793) (-14.4975, -20.8002) (-14.4975, -20.5705) knots 0 0 0 1 2 2 2
  spline S189 degree 2 poles (-14.4975, -20.5705) (-14.4975, -20.3877) (-14.6778, -20.1605) (-14.873, -20.1037) knots 0 0 0 1 2 2 2
  spline S190 degree 2 poles (-14.873, -20.1037) (-15.0138, -20.0641) (-15.2484, -20.0098) (-15.4238, -19.9653) knots 0 0 0 1 2 2 2
  spline S191 degree 2 poles (-15.4238, -19.9653) (-15.5819, -19.9234) (-15.8313, -19.7974) (-15.9277, -19.6961) knots 0 0 0 1 2 2 2
  spline S192 degree 2 poles (-15.9277, -19.6961) (-16.0215, -19.5948) (-16.1253, -19.3231) (-16.1253, -19.1453) knots 0 0 0 1 2 2 2
  spline S193 degree 2 poles (-16.1253, -19.1453) (-16.1253, -18.7748) (-15.5473, -18.2734) (-15.1002, -18.2734) knots 0 0 0 1 2 2 2
  spline S194 degree 2 poles (-15.1002, -18.2734) (-14.8433, -18.2734) (-14.3889, -18.3747) (-14.1937, -18.471) knots 0 0 0 1 2 2 2
  line L150 (-14.1937, -18.471) -> (-14.1937, -18.9551)
  line L151 (-14.1937, -18.9551) -> (-14.2234, -18.9551)
  spline S195 degree 2 poles (-14.2234, -18.9551) (-14.3691, -18.8217) (-14.8236, -18.6241) (-15.073, -18.6241) knots 0 0 0 1 2 2 2
  spline S196 degree 2 poles (-15.073, -18.6241) (-15.3546, -18.6241) (-15.7029, -18.8884) (-15.7029, -19.1033) knots 0 0 0 1 2 2 2
  spline S197 degree 2 poles (-15.7029, -19.1033) (-15.7029, -19.296) (-15.4979, -19.5257) (-15.3052, -19.5776) knots 0 0 0 1 2 2 2
  spline S198 degree 2 poles (-15.3052, -19.5776) (-15.1768, -19.6121) (-14.8038, -19.7011) (-14.6803, -19.7381) knots 0 0 0 1 2 2 2
  spline S199 degree 2 poles (-14.6803, -19.7381) (-14.3666, -19.8344) (-14.0752, -20.2222) (-14.0752, -20.5063) knots 0 0 0 1 2 2 2
  spline S200 degree 2 poles (-14.0752, -20.5063) (-14.0752, -20.6866) (-14.2209, -21.0324) (-14.3518, -21.1534) knots 0 0 0 1 2 2 2
  spline S201 degree 2 poles (-14.3518, -21.1534) (-14.4975, -21.2868) (-14.868, -21.4301) (-15.1471, -21.4301) knots 0 0 0 1 2 2 2
  spline S202 degree 2 poles (-11.7756, -20.1704) (-11.7756, -20.7434) (-12.3215, -21.4202) (-12.7389, -21.4202) knots 0 0 0 1 2 2 2
  spline S203 degree 2 poles (-12.7389, -21.4202) (-12.9093, -21.4202) (-13.1711, -21.3411) (-13.307, -21.2596) knots 0 0 0 1 2 2 2
  line L152 (-13.307, -21.2596) -> (-13.307, -22.218)
  line L153 (-13.307, -22.218) -> (-13.6923, -22.218)
  line L154 (-13.6923, -22.218) -> (-13.6923, -19.0885)
  line L155 (-13.6923, -19.0885) -> (-13.307, -19.0885)
  line L156 (-13.307, -19.0885) -> (-13.307, -19.3281)
  spline S204 degree 2 poles (-13.307, -19.3281) (-13.1637, -19.1972) (-12.813, -19.0243) (-12.608, -19.0243) knots 0 0 0 1 2 2 2
  spline S205 degree 2 poles (-12.608, -19.0243) (-12.2152, -19.0243) (-11.7756, -19.6467) (-11.7756, -20.1704) knots 0 0 0 1 2 2 2
  spline S206 degree 2 poles (-12.1733, -20.2148) (-12.1733, -19.8221) (-12.4227, -19.3898) (-12.7018, -19.3898) knots 0 0 0 1 2 2 2
  spline S207 degree 2 poles (-12.7018, -19.3898) (-12.8649, -19.3898) (-13.1711, -19.5356) (-13.307, -19.6492) knots 0 0 0 1 2 2 2
  line L157 (-13.307, -19.6492) -> (-13.307, -20.9484)
  spline S208 degree 2 poles (-13.307, -20.9484) (-13.1563, -21.02) (-12.9414, -21.0744) (-12.8031, -21.0744) knots 0 0 0 1 2 2 2
  spline S209 degree 2 poles (-12.8031, -21.0744) (-12.5042, -21.0744) (-12.1733, -20.6347) (-12.1733, -20.2148) knots 0 0 0 1 2 2 2
  line L158 (-10.1627, -19.501) -> (-10.1824, -19.501)
  spline S210 degree 2 poles (-10.1824, -19.501) (-10.2269, -19.4886) (-10.3232, -19.4837) (-10.3899, -19.4837) knots 0 0 0 1 2 2 2
  spline S211 degree 2 poles (-10.3899, -19.4837) (-10.5455, -19.4837) (-10.8518, -19.6195) (-10.9901, -19.7529) knots 0 0 0 1 2 2 2
  line L159 (-10.9901, -19.7529) -> (-10.9901, -21.3757)
  line L160 (-10.9901, -21.3757) -> (-11.3754, -21.3757)
  line L161 (-11.3754, -21.3757) -> (-11.3754, -19.0885)
  line L162 (-11.3754, -19.0885) -> (-10.9901, -19.0885)
  line L163 (-10.9901, -19.0885) -> (-10.9901, -19.4294)
  spline S212 degree 2 poles (-10.9901, -19.4294) (-10.7802, -19.2416) (-10.4665, -19.0885) (-10.3183, -19.0885) knots 0 0 0 1 2 2 2
  spline S213 degree 2 poles (-10.3183, -19.0885) (-10.259, -19.0885) (-10.1997, -19.0934) (-10.1627, -19.1008) knots 0 0 0 1 2 2 2
  line L164 (-10.1627, -19.1008) -> (-10.1627, -19.501)
  line L165 (-9.4711, -21.3757) -> (-9.8564, -21.3757)
  line L166 (-9.8564, -21.3757) -> (-9.8564, -19.0885)
  line L167 (-9.8564, -19.0885) -> (-9.4711, -19.0885)
  line L168 (-9.4711, -19.0885) -> (-9.4711, -21.3757)
  line L169 (-9.4439, -18.7081) -> (-9.8811, -18.7081)
  line L170 (-9.8811, -18.7081) -> (-9.8811, -18.308)
  line L171 (-9.8811, -18.308) -> (-9.4439, -18.308)
  line L172 (-9.4439, -18.308) -> (-9.4439, -18.7081)
  line L173 (-7.1097, -21.3757) -> (-7.495, -21.3757)
  line L174 (-7.495, -21.3757) -> (-7.495, -20.0716)
  spline S214 degree 2 poles (-7.495, -20.0716) (-7.495, -19.9135) (-7.5247, -19.6418) (-7.5691, -19.5603) knots 0 0 0 1 2 2 2
  spline S215 degree 2 poles (-7.5691, -19.5603) (-7.6161, -19.4738) (-7.784, -19.3898) (-7.9273, -19.3898) knots 0 0 0 1 2 2 2
  spline S216 degree 2 poles (-7.9273, -19.3898) (-8.0706, -19.3898) (-8.3744, -19.543) (-8.5201, -19.6665) knots 0 0 0 1 2 2 2
  line L175 (-8.5201, -19.6665) -> (-8.5201, -21.3757)
  line L176 (-8.5201, -21.3757) -> (-8.9054, -21.3757)
  line L177 (-8.9054, -21.3757) -> (-8.9054, -19.0885)
  line L178 (-8.9054, -19.0885) -> (-8.5201, -19.0885)
  line L179 (-8.5201, -19.0885) -> (-8.5201, -19.3429)
  spline S217 degree 2 poles (-8.5201, -19.3429) (-8.3472, -19.1873) (-8.0137, -19.0243) (-7.826, -19.0243) knots 0 0 0 1 2 2 2
  spline S218 degree 2 poles (-7.826, -19.0243) (-7.4901, -19.0243) (-7.1097, -19.4689) (-7.1097, -19.8912) knots 0 0 0 1 2 2 2
  line L180 (-7.1097, -19.8912) -> (-7.1097, -21.3757)
  spline S219 degree 2 poles (-6.4873, -21.7413) (-6.4478, -21.7586) (-6.2971, -21.8129) (-6.2008, -21.8351) knots 0 0 0 1 2 2 2
  spline S220 degree 2 poles (-6.2008, -21.8351) (-6.0945, -21.8623) (-5.9142, -21.8944) (-5.808, -21.8944) knots 0 0 0 1 2 2 2
  spline S221 degree 2 poles (-5.808, -21.8944) (-5.6302, -21.8944) (-5.3832, -21.8006) (-5.314, -21.7166) knots 0 0 0 1 2 2 2
  spline S222 degree 2 poles (-5.314, -21.7166) (-5.2473, -21.6326) (-5.1955, -21.4128) (-5.1955, -21.272) knots 0 0 0 1 2 2 2
  line L181 (-5.1955, -21.272) -> (-5.1955, -21.0719)
  spline S223 degree 2 poles (-5.1955, -21.0719) (-5.3511, -21.2078) (-5.6499, -21.3362) (-5.8747, -21.3362) knots 0 0 0 1 2 2 2
  spline S224 degree 2 poles (-5.8747, -21.3362) (-6.265, -21.3362) (-6.7269, -20.7558) (-6.7269, -20.2099) knots 0 0 0 1 2 2 2
  spline S225 degree 2 poles (-6.7269, -20.2099) (-6.7269, -19.9258) (-6.5663, -19.4862) (-6.4329, -19.3306) knots 0 0 0 1 2 2 2
  spline S226 degree 2 poles (-6.4329, -19.3306) (-6.3045, -19.1848) (-5.9513, -19.0243) (-5.7636, -19.0243) knots 0 0 0 1 2 2 2
  spline S227 degree 2 poles (-5.7636, -19.0243) (-5.5857, -19.0243) (-5.3264, -19.1082) (-5.1955, -19.1848) knots 0 0 0 1 2 2 2
  line L182 (-5.1955, -19.1848) -> (-5.1732, -19.0885)
  line L183 (-5.1732, -19.0885) -> (-4.8101, -19.0885)
  line L184 (-4.8101, -19.0885) -> (-4.8101, -21.1139)
  spline S228 degree 2 poles (-4.8101, -21.1139) (-4.8101, -21.6968) (-5.3165, -22.2402) (-5.8377, -22.2402) knots 0 0 0 1 2 2 2
  spline S229 degree 2 poles (-5.8377, -22.2402) (-6.0056, -22.2402) (-6.3564, -22.1859) (-6.507, -22.1414) knots 0 0 0 1 2 2 2
  line L185 (-6.507, -22.1414) -> (-6.507, -21.7413)
  line L186 (-6.507, -21.7413) -> (-6.4873, -21.7413)
  line L187 (-5.1955, -20.7558) -> (-5.1955, -19.4985)
  spline S230 degree 2 poles (-5.1955, -19.4985) (-5.3387, -19.4294) (-5.5808, -19.3701) (-5.7018, -19.3701) knots 0 0 0 1 2 2 2
  spline S231 degree 2 poles (-5.7018, -19.3701) (-5.9933, -19.3701) (-6.3292, -19.7999) (-6.3292, -20.2025) knots 0 0 0 1 2 2 2
  spline S232 degree 2 poles (-6.3292, -20.2025) (-6.3292, -20.5828) (-6.0748, -20.9805) (-5.7883, -20.9805) knots 0 0 0 1 2 2 2
  spline S233 degree 2 poles (-5.7883, -20.9805) (-5.6376, -20.9805) (-5.3214, -20.862) (-5.1955, -20.7558) knots 0 0 0 1 2 2 2
  line L188 (-1.8832, -20.2272) -> (-3.0367, -20.2272)
  line L189 (-3.0367, -20.2272) -> (-3.0367, -19.8567)
  line L190 (-3.0367, -19.8567) -> (-1.8832, -19.8567)
  line L191 (-1.8832, -19.8567) -> (-1.8832, -20.2272)
  line L192 (1.7404, -18.6883) -> (0.3226, -18.6883)
  line L193 (0.3226, -18.6883) -> (0.3226, -19.5479)
  line L194 (0.3226, -19.5479) -> (1.6811, -19.5479)
  line L195 (1.6811, -19.5479) -> (1.6811, -19.9085)
  line L196 (1.6811, -19.9085) -> (0.3226, -19.9085)
  line L197 (0.3226, -19.9085) -> (0.3226, -21.3757)
  line L198 (0.3226, -21.3757) -> (-0.0825, -21.3757)
  line L199 (-0.0825, -21.3757) -> (-0.0825, -18.3277)
  line L200 (-0.0825, -18.3277) -> (1.7404, -18.3277)
  line L201 (1.7404, -18.3277) -> (1.7404, -18.6883)
  spline S234 degree 2 poles (3.3483, -21.1337) (3.3014, -21.1682) (3.1433, -21.2917) (3.0692, -21.3288) knots 0 0 0 1 2 2 2
  spline S235 degree 2 poles (3.0692, -21.3288) (2.9679, -21.3831) (2.7778, -21.4399) (2.6049, -21.4399) knots 0 0 0 1 2 2 2
  spline S236 degree 2 poles (2.6049, -21.4399) (2.4641, -21.4399) (2.2097, -21.3337) (2.1133, -21.2374) knots 0 0 0 1 2 2 2
  spline S237 degree 2 poles (2.1133, -21.2374) (2.0219, -21.1435) (1.9108, -20.8669) (1.9108, -20.7138) knots 0 0 0 1 2 2 2
  spline S238 degree 2 poles (1.9108, -20.7138) (1.9108, -20.4766) (2.1109, -20.1407) (2.3282, -20.0444) knots 0 0 0 1 2 2 2
  spline S239 degree 2 poles (2.3282, -20.0444) (2.5209, -19.9555) (3.0445, -19.8888) (3.3483, -19.8715) knots 0 0 0 1 2 2 2
  line L202 (3.3483, -19.8715) -> (3.3483, -19.7974)
  spline S240 degree 2 poles (3.3483, -19.7974) (3.3483, -19.664) (3.2668, -19.4985) (3.1927, -19.4516) knots 0 0 0 1 2 2 2
  spline S241 degree 2 poles (3.1927, -19.4516) (3.1186, -19.4047) (2.9062, -19.375) (2.7926, -19.375) knots 0 0 0 1 2 2 2
  spline S242 degree 2 poles (2.7926, -19.375) (2.6592, -19.375) (2.2986, -19.4541) (2.1183, -19.5306) knots 0 0 0 1 2 2 2
  line L203 (2.1183, -19.5306) -> (2.096, -19.5306)
  line L204 (2.096, -19.5306) -> (2.096, -19.1379)
  spline S243 degree 2 poles (2.096, -19.1379) (2.2022, -19.1082) (2.5999, -19.0341) (2.795, -19.0341) knots 0 0 0 1 2 2 2
  spline S244 degree 2 poles (2.795, -19.0341) (3.0322, -19.0341) (3.3557, -19.1082) (3.4842, -19.2046) knots 0 0 0 1 2 2 2
  spline S245 degree 2 poles (3.4842, -19.2046) (3.6102, -19.2984) (3.7337, -19.5973) (3.7337, -19.8122) knots 0 0 0 1 2 2 2
  line L205 (3.7337, -19.8122) -> (3.7337, -21.3757)
  line L206 (3.7337, -21.3757) -> (3.3483, -21.3757)
  line L207 (3.3483, -21.3757) -> (3.3483, -21.1337)
  line L208 (3.3483, -20.8126) -> (3.3483, -20.1778)
  spline S246 degree 2 poles (3.3483, -20.1778) (3.21, -20.1901) (2.7926, -20.2321) (2.6617, -20.2716) knots 0 0 0 1 2 2 2
  spline S247 degree 2 poles (2.6617, -20.2716) (2.5085, -20.3186) (2.3085, -20.5137) (2.3085, -20.6866) knots 0 0 0 1 2 2 2
  spline S248 degree 2 poles (2.3085, -20.6866) (2.3085, -20.8842) (2.5308, -21.0843) (2.7432, -21.0843) knots 0 0 0 1 2 2 2
  spline S249 degree 2 poles (2.7432, -21.0843) (2.9235, -21.0843) (3.2199, -20.9287) (3.3483, -20.8126) knots 0 0 0 1 2 2 2
  line L209 (4.6673, -21.3757) -> (4.282, -21.3757)
  line L210 (4.282, -21.3757) -> (4.282, -18.1919)
  line L211 (4.282, -18.1919) -> (4.6673, -18.1919)
  line L212 (4.6673, -18.1919) -> (4.6673, -21.3757)
  line L213 (5.6257, -21.3757) -> (5.2404, -21.3757)
  line L214 (5.2404, -21.3757) -> (5.2404, -18.1919)
  line L215 (5.2404, -18.1919) -> (5.6257, -18.1919)
  line L216 (5.6257, -18.1919) -> (5.6257, -21.3757)
  line L217 (9.3233, -21.3757) -> (7.4436, -21.3757)
  line L218 (7.4436, -21.3757) -> (7.4436, -20.9435)
  spline S250 degree 2 poles (7.4436, -20.9435) (7.6462, -20.7533) (8.0068, -20.4001) (8.1797, -20.2099) knots 0 0 0 1 2 2 2
  spline S251 degree 2 poles (8.1797, -20.2099) (8.528, -19.827) (8.7824, -19.3676) (8.7824, -19.1231) knots 0 0 0 1 2 2 2
  spline S252 degree 2 poles (8.7824, -19.1231) (8.7824, -18.9946) (8.7033, -18.802) (8.6317, -18.7402) knots 0 0 0 1 2 2 2
  spline S253 degree 2 poles (8.6317, -18.7402) (8.5601, -18.6785) (8.3723, -18.6167) (8.2587, -18.6167) knots 0 0 0 1 2 2 2
  spline S254 degree 2 poles (8.2587, -18.6167) (8.15, -18.6167) (7.9277, -18.6711) (7.8265, -18.713) knots 0 0 0 1 2 2 2
  spline S255 degree 2 poles (7.8265, -18.713) (7.74, -18.7476) (7.5795, -18.8464) (7.5301, -18.881) knots 0 0 0 1 2 2 2
  line L219 (7.5301, -18.881) -> (7.5078, -18.881)
  line L220 (7.5078, -18.881) -> (7.5078, -18.4463)
  spline S256 degree 2 poles (7.5078, -18.4463) (7.6338, -18.3845) (8.0858, -18.2635) (8.2884, -18.2635) knots 0 0 0 1 2 2 2
  spline S257 degree 2 poles (8.2884, -18.2635) (8.7157, -18.2635) (9.1973, -18.7155) (9.1973, -19.1008) knots 0 0 0 1 2 2 2
  spline S258 degree 2 poles (9.1973, -19.1008) (9.1973, -19.2812) (9.1133, -19.5825) (9.0392, -19.7109) knots 0 0 0 1 2 2 2
  spline S259 degree 2 poles (9.0392, -19.7109) (8.9651, -19.8443) (8.7503, -20.1061) (8.6317, -20.2321) knots 0 0 0 1 2 2 2
  spline S260 degree 2 poles (8.6317, -20.2321) (8.439, -20.4421) (7.9673, -20.8916) (7.8265, -21.0225) knots 0 0 0 1 2 2 2
  line L221 (7.8265, -21.0225) -> (9.3233, -21.0225)
  line L222 (9.3233, -21.0225) -> (9.3233, -21.3757)
  spline S261 degree 2 poles (11.6278, -19.8517) (11.6278, -20.6718) (11.1511, -21.4399) (10.6546, -21.4399) knots 0 0 0 1 2 2 2
  spline S262 degree 2 poles (10.6546, -21.4399) (10.1508, -21.4399) (9.679, -20.6569) (9.679, -19.8542) knots 0 0 0 1 2 2 2
  spline S263 degree 2 poles (9.679, -19.8542) (9.679, -19.0292) (10.1557, -18.266) (10.6546, -18.266) knots 0 0 0 1 2 2 2
  spline S264 degree 2 poles (10.6546, -18.266) (11.1561, -18.266) (11.6278, -19.0564) (11.6278, -19.8517) knots 0 0 0 1 2 2 2
  spline S265 degree 2 poles (11.1042, -20.7805) (11.1635, -20.6298) (11.2129, -20.1654) (11.2129, -19.8517) knots 0 0 0 1 2 2 2
  spline S266 degree 2 poles (11.2129, -19.8517) (11.2129, -19.538) (11.1635, -19.0761) (11.1017, -18.9205) knots 0 0 0 1 2 2 2
  spline S267 degree 2 poles (11.1017, -18.9205) (11.04, -18.7649) (10.8251, -18.6044) (10.6546, -18.6044) knots 0 0 0 1 2 2 2
  spline S268 degree 2 poles (10.6546, -18.6044) (10.4842, -18.6044) (10.2644, -18.7649) (10.2002, -18.9255) knots 0 0 0 1 2 2 2
  spline S269 degree 2 poles (10.2002, -18.9255) (10.1384, -19.0811) (10.0939, -19.5553) (10.0939, -19.8542) knots 0 0 0 1 2 2 2
  spline S270 degree 2 poles (10.0939, -19.8542) (10.0939, -20.1753) (10.1335, -20.6051) (10.1977, -20.773) knots 0 0 0 1 2 2 2
  spline S271 degree 2 poles (10.1977, -20.773) (10.257, -20.9311) (10.4768, -21.1016) (10.6546, -21.1016) knots 0 0 0 1 2 2 2
  spline S272 degree 2 poles (10.6546, -21.1016) (10.8226, -21.1016) (11.0424, -20.941) (11.1042, -20.7805) knots 0 0 0 1 2 2 2
  line L223 (13.8978, -21.3757) -> (12.0181, -21.3757)
  line L224 (12.0181, -21.3757) -> (12.0181, -20.9435)
  spline S273 degree 2 poles (12.0181, -20.9435) (12.2206, -20.7533) (12.5813, -20.4001) (12.7542, -20.2099) knots 0 0 0 1 2 2 2
  spline S274 degree 2 poles (12.7542, -20.2099) (13.1024, -19.827) (13.3568, -19.3676) (13.3568, -19.1231) knots 0 0 0 1 2 2 2
  spline S275 degree 2 poles (13.3568, -19.1231) (13.3568, -18.9946) (13.2778, -18.802) (13.2062, -18.7402) knots 0 0 0 1 2 2 2
  spline S276 degree 2 poles (13.2062, -18.7402) (13.1345, -18.6785) (12.9468, -18.6167) (12.8332, -18.6167) knots 0 0 0 1 2 2 2
  spline S277 degree 2 poles (12.8332, -18.6167) (12.7245, -18.6167) (12.5022, -18.6711) (12.4009, -18.713) knots 0 0 0 1 2 2 2
  spline S278 degree 2 poles (12.4009, -18.713) (12.3145, -18.7476) (12.1539, -18.8464) (12.1045, -18.881) knots 0 0 0 1 2 2 2
  line L225 (12.1045, -18.881) -> (12.0823, -18.881)
  line L226 (12.0823, -18.881) -> (12.0823, -18.4463)
  spline S279 degree 2 poles (12.0823, -18.4463) (12.2083, -18.3845) (12.6603, -18.2635) (12.8628, -18.2635) knots 0 0 0 1 2 2 2
  spline S280 degree 2 poles (12.8628, -18.2635) (13.2901, -18.2635) (13.7718, -18.7155) (13.7718, -19.1008) knots 0 0 0 1 2 2 2
  spline S281 degree 2 poles (13.7718, -19.1008) (13.7718, -19.2812) (13.6878, -19.5825) (13.6137, -19.7109) knots 0 0 0 1 2 2 2
  spline S282 degree 2 poles (13.6137, -19.7109) (13.5396, -19.8443) (13.3247, -20.1061) (13.2062, -20.2321) knots 0 0 0 1 2 2 2
  spline S283 degree 2 poles (13.2062, -20.2321) (13.0135, -20.4421) (12.5417, -20.8916) (12.4009, -21.0225) knots 0 0 0 1 2 2 2
  line L227 (12.4009, -21.0225) -> (13.8978, -21.0225)
  line L228 (13.8978, -21.0225) -> (13.8978, -21.3757)
  line L229 (16.2665, -20.3284) -> (15.9034, -20.3284)
  line L230 (15.9034, -20.3284) -> (15.9034, -21.3757)
  line L231 (15.9034, -21.3757) -> (15.5107, -21.3757)
  line L232 (15.5107, -21.3757) -> (15.5107, -20.3284)